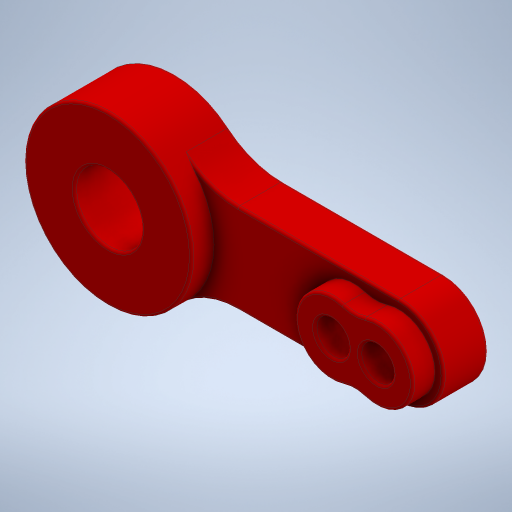
# Autodesk Inventor part: 25T M3
Saved by Autodesk Inventor 2024 (Build 280153000, 153)
## iProperties
Created: 2024-04-17
Part Number: 25T M3
Material: Generic
Document SubType Name: Modeling
Designer: compu
Density: 1 g/cm^3
Appearance: Default
Author: compu
Autodesk Inventor part; units mm, degrees
ref_plane "YZ Plane" through (0, 0, 0) normal (1, 0, 0) x (0, 1, 0)
ref_plane "XZ Plane" through (0, 0, 0) normal (0, 1, 0) x (-1, 0, 0)
ref_plane "XY Plane" through (0, 0, 0) normal (0, 0, 1) x (1, 0, 0)
sketch "Sketch1" plane through (0, 0, 0) normal (0, 0, 1) x (1, 0, 0)
  circle A0 centre (0, 0) radius 7.5
  circle A1 centre (24, 0) radius 1.5
  line L0 (-14.6, 0) -> (35.1, 0) projected
  line L1 (0, -16.1) -> (0, 16.1) projected
  line L2 (24, 4) -> (6.3443, 4)
  line L3 (24, -4) -> (6.3443, -4)
  arc A2 (9.6307, -4) -> (4.8153, -5.75) centre (9.6307, -11.5) ccw
  arc A3 (24, -4) -> (24, 4) centre (24, 0) ccw
  circle A4 centre (20, 0) radius 1.5
  arc A5 (21, 3.0923) -> (21, -3.0923) centre (20, 0) ccw
  arc A6 (21, 3.0923) -> (23, 3.0923) centre (22, 6.1847) ccw
  arc A7 (23, -3.0923) -> (21, -3.0923) centre (22, -6.1847) ccw
  arc A8 (23, -3.0923) -> (23, 3.0923) centre (24, 0) ccw
  arc A9 (4.8153, 5.75) -> (9.6307, 4) centre (9.6307, 11.5) ccw
  circle A10 centre (0, 0) radius 3
  dimension "d0" = 15
  dimension "d1" = 3
  dimension "d2" = 24
  dimension "d7" = 3
  dimension "d8" = 20
  dimension "d9" = 6.5
  dimension "d10" = 6.5
  dimension "d11" = 6.5
  dimension "d12" = 4
  dimension "d13" = 3.25
  dimension "d14" = 15
  dimension "d15" = 15
  dimension "d16" = 6
  constraints: 18 point on circle, 11 centre point, 10 tangent, 5 coincident, 4 end point, 4 point on line, 2 horizontal
  measures "d0" diameter of A0
  measures "d1" diameter of A1
  measures "d2" distance of A1.centre point (0, 0)
  measures "d7" diameter of A4
  measures "d8" distance of point (0, 0) A4.centre
  measures "d9" diameter of A5
  measures "d10" diameter of A6
  measures "d11" diameter of A7
  measures "d12" radius of A3
  measures "d13" radius of A8
  measures "d14" diameter of A2
  measures "d15" diameter of A9
  measures "d16" diameter of A10
extrude "Extrusion1" add sketch "Sketch1" along normal blind 6 contours L0 A10 L1 A0 | A0 L1 A10 L0 | A5 A6 A8 L0 A1 A4 | L0 A4 A1 A8 A7 A5 | A10 L0 A0 L1 | L1 A0 L0 A10
extrude "Extrusion2" add sketch "Sketch1" along normal blind 4 contours L0 A5 A7 A8 A3 L3 A0 | A0 L2 A3 L0 A8 A6 A5 | A0 A9 L2 | L3 A2 A0
fillet "Fillet1" radius 0.2 1 edges at (-7.5, 0, 6)
fillet "Fillet2" radius 0.2 20 edges at (-3, 0, 6) (16.8153, 4, 4) (28, 0, 4) (16.8153, -4, 4) (7.0689, -4.4511, 4) (7.0689, 4.4511, 4) (22, 2.9347, 6) (16.75, 0, 6) (22, -2.9347, 6) (27.25, 0, 6) (18.5, 0, 6) (7.0689, 4.4511, 0) (-7.5, 0, 0) (7.0689, -4.4511, 0) (16.8153, -4, 0) (28, 0, 0) (16.8153, 4, 0) (18.5, 0, 0) (-3, 0, 0) (22.5, 0, 0)
fillet "Fillet3" radius 0.2 1 edges at (22.5, 0, 6)
body "Solid1"
